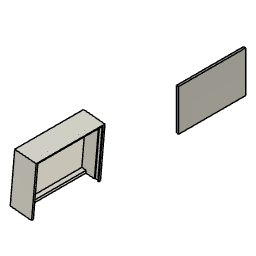
Configuration cool v3 (Autodesk Fusion 360 design; units mm, degrees)
Autodesk Fusion 360 part; units mm, degrees
note: some values were not read from the file. Set by a fixed rule: which sketch regions a step uses.
sketch "Sketch1" plane through (0, 0, 0) normal (1, 0, 0) x (0, 1, 0)
  line L0 (0, 0) -> (80, 0)
  line L1 (0, 0) -> (0, 60)
  line L2 (0, 60) -> (80, 60)
  line L3 (80, 60) -> (80, 0)
  dimension "d1" = 80
  constraint coincident L0.start L1.start
  constraint horizontal L0
  constraint perpendicular L0 L1
  constraint perpendicular L1 L2
  constraint perpendicular L0 L3
  measures "d1" distance of L0.start L0.end
extrude "Extrude1" add sketch "Sketch1" along normal blind 10 makes body 1
sketch "Sketch2" plane through (10, 0, 0) normal (1, 0, 0) x (0, 1, 0)
  line L0 (0, 0) -> (80, 0)
  line L1 (80, 0) -> (80, 60)
  line L2 (80, 60) -> (0, 60)
  line L3 (0, 60) -> (0, 0)
  line L4 (0, 60) -> (80, 60)
  line L5 (80, 0) -> (38, 0)
  line L6 (38, 58.7474) -> (2, 58.7474)
  line L7 (2, 58.7474) -> (2, 0)
  line L8 (0, 0) -> (2, 0)
  line L9 (38, 58.7474) -> (38, 0)
  constraint coincident L2.end L3.start
  constraint coincident L1.end L2.start
  constraint coincident L0.end L1.start
  constraint coincident L0 L5.end
  constraint perpendicular L1 L5
  constraint perpendicular L1 L6
  constraint coincident L0 L7.end
  constraint perpendicular L0 L7
  constraint coincident L0.start L3.end
  constraint perpendicular L5 L9
extrude "Extrude2" add sketch "Sketch2" along normal blind 15 contours L0 L1 L2 L3 L4 L5 L6 L7 L8 L9 bodies 1
sketch "Sketch3" plane through (10, 0, 0) normal (1, 0, 0) x (0, 1, 0)
  line L0 (2, 58.7474) -> (2, 0)
  line L1 (2, 0) -> (38, 0)
  line L2 (2, 0) -> (38, 0)
  line L3 (38, 2.9429) -> (2, 2.9429)
  line L4 (2, 0) -> (2, 2.9429)
  line L5 (38, 0) -> (38, 2.9429)
  line L6 (38, 0) -> (38, 58.7474)
  line L7 (38, 58.7474) -> (2, 58.7474)
  constraint coincident L0.end L1.start
  constraint coincident L1.end L2.end
  constraint coincident L0 L3.end
  constraint perpendicular L0 L3
  constraint perpendicular L3 L5
extrude "Extrude3" add sketch "Sketch3" along normal blind 5 contours L0 L1 L2 L3 L4 L5 L6 bodies 1
sketch "Sketch4" plane through (10, 0, 0) normal (1, 0, 0) x (0, 1, 0)
  line L0 (2, 2.9429) -> (38, 2.9429)
  line L1 (2, 58.7474) -> (2, 2.9429)
  line L2 (33.2817, -3.5012) -> (111.2817, -3.5012)
  line L3 (111.2817, -3.5012) -> (111.2817, 44.4988)
  line L4 (111.2817, 44.4988) -> (33.2817, 44.4988)
  line L5 (33.2817, 44.4988) -> (33.2817, -3.5012)
  line L6 (38, 2.9429) -> (38, 58.7474)
  line L7 (38, 58.7474) -> (2, 58.7474)
  dimension "d8" = 78
  dimension "d9" = 48
  constraint perpendicular L2 L3
  constraint perpendicular L3 L4
  constraint perpendicular L2 L5
  measures "d8" distance of L2.start L2.end
  measures "d9" distance of L2.end L3.end
extrude "Extrude4" add sketch "Sketch4" along normal blind 2 separate body contours L0 L4 L5 L6 | L0 L2 L3 L4 L5 L6 makes body 2
sketch "Sketch5" plane through (12, 0, 0) normal (1, 0, 0) x (0, 1, 0)
  line L0 (33.2817, 44.4988) -> (33.2817, -3.5012)
  line L1 (33.2817, -3.5012) -> (111.2817, -3.5012)
  line L2 (111.2817, -3.5012) -> (111.2817, 44.4988)
  line L3 (111.2817, 44.4988) -> (33.2817, 44.4988)
move_body "Move1" bodies 2 to x (1, 0, 0) y (0, 1, 0) z (0, 0, 1) at (15, -48, 2)
move_body "Move2" bodies 2 to x (1, 0, 0) y (0, 1, 0) z (0, 0, 1) at (-6, 0, 0)
sketch "Sketch6" plane through (21, 0, 0) normal (1, 0, 0) x (0, 1, 0)
  line L0 (-14.7183, 46.4988) -> (-14.7183, -1.5012)
  line L1 (-14.7183, -1.5012) -> (63.2817, -1.5012)
  line L2 (63.2817, -1.5012) -> (63.2817, 46.4988)
  line L3 (63.2817, 46.4988) -> (-14.7183, 46.4988)
move_body "Move3" bodies 2 to x (1, 0, 0) y (0, 1, 0) z (0, 0, 1) at (18, 0, 0)
sketch "Sketch7" plane through (39, 0, 0) normal (1, 0, 0) x (0, 1, 0)
  line L0 (-14.7183, 46.4988) -> (-14.7183, -1.5012)
  line L1 (-14.7183, -1.5012) -> (63.2817, -1.5012)
  line L2 (63.2817, -1.5012) -> (63.2817, 46.4988)
  line L3 (63.2817, 46.4988) -> (-14.7183, 46.4988)
sketch "Sketch8" plane through (39, 0, 0) normal (1, 0, 0) x (0, 1, 0)
  line L0 (-14.7183, 46.4988) -> (-14.7183, -1.5012)
  line L1 (-14.7183, -1.5012) -> (63.2817, -1.5012)
  line L2 (63.2817, -1.5012) -> (63.2817, 46.4988)
  line L3 (63.2817, 46.4988) -> (-14.7183, 46.4988)
move_body "Move4" bodies 2 to x (1, 0, 0) y (0, 1, 0) z (0, 0, 1) at (-1.5428, 1.8094, 0.4773)
move_body "Move5" bodies 2 to x (1, 0, 0) y (0, 1, 0) z (0, 0, 1) at (0, 10, 0)
move_body "Move6" bodies 2 to x (1, 0, 0) y (0, 1, 0) z (0, 0, 1) at (-15, 0, 0)
move_body "Move7" bodies 2 to x (1, 0, 0) y (0, 1, 0) z (0, 0, 1) at (0, -12, 0)
move_body "Move8" bodies 2 to x (1, 0, 0) y (0, 1, 0) z (0, 0, 1) at (10, 0, 0)
move_body "Move9" bodies 2 to x (1, 0, 0) y (0, 1, 0) z (0, 0, 1) at (0, 15, 5)
move_body "Move10" bodies 2 to x (1, 0, 0) y (0, 1, 0) z (0, 0, 1) at (0.5173, -18.9965, -0.6609)
move_body "Move11" bodies 2 to x (1, 0, 0) y (0, 1, 0) z (0, 0, 1) at (-13, 0, 0)
move_body "Move12" bodies 2 to x (1, 0, 0) y (0, 1, 0) z (0, 0, 1) at (0, 4, 0)
move_body "Move13" bodies 2 to x (1, 0, 0) y (0, 1, 0) z (0, 0, 1) at (10, 0, 0)
move_body "Move14" bodies 2 to x (1, 0, 0) y (0, 1, 0) z (0, 0, 1) at (0, 1, 0)
move_body "Move15" bodies 2 to x (1, 0, 0) y (0, 1, 0) z (0, 0, 1) at (21.2708, 41.4828, -21.4534)
move_body "Move16" bodies 2 to x (1, 0, 0) y (0, 1, 0) z (0, 0, 1) at (3.3836, 8.6688, 28.5327)
move_body "Move17" bodies 2 to x (1, 0, 0) y (0, 1, 0) z (0, 0, 1) at (-38.2468, 34.7717, -10.8051)
extrude "Extrude6" cut 1 faces at (16.6667, 38, 40.1459) along direction (0, 1, 0) blind 40 on bodies 1 bodies 1
extrude "Extrude7" add 1 faces at (25, 0.6667, 39.5825) along direction (1, 0, 0) blind 5 on bodies 1 bodies 1
sketch "Sketch10" plane through (0, 78, 0) normal (0, -1, 0) x (1, 0, 0)
  line L0 (15, 2.9429) -> (15, 0)
  line L1 (15, 0) -> (30, 0)
  line L2 (30, 0) -> (30, 58.7474)
  line L3 (30, 58.7474) -> (10, 58.7474)
  line L4 (10, 58.7474) -> (10, 2.9429)
  line L5 (10, 2.9429) -> (15, 2.9429)
move_body "Move18" bodies 2 to x (1, 0, 0) y (0, 1, 0) z (0, 0, 1) at (-1.1862, -16.387, -16.5072)
move_body "Move19" bodies 2 to x (1, 0, 0) y (0, 1, 0) z (0, 0, 1) at (16.0791, -7.3134, -20.0229)
move_body "Move20" bodies 2 to x (1, 0, 0) y (0, 1, 0) z (0, 0, 1) at (3.6083, -61.8453, 40.1901)
move_body "Move21" bodies 2 to x (1, 0, 0) y (0, 1, 0) z (0, 0, 1) at (0, 62.0564, 0.6442)
move_body "Move22" bodies 2 to x (1, 0, 0) y (0, 1, 0) z (0, 0, 1) at (0, 24.1549, -0.0402)
extrude "Extrude9" cut 1 faces at (0, 53.3333, 20) along direction (1, 0, 0) blind 5 on bodies 1 bodies 1
move_body "Move23" bodies 2 to x (1, 0, 0) y (0, 1, 0) z (0, 0, 1) at (29.6008, -117.5704, 12.6132)
move_face "MoveFace2" by (0.4671, 2.2152, 0.1877) 1 faces at (64.4841, -19.887, 48.4665) on bodies 2
move_body "Move24" bodies 2 to x (1, 0, 0) y (0, 1, 0) z (0, 0, 1) at (7.9958, 36.4984, 0.1207)
move_body "Move25" bodies 2 to x (1, 0, 0) y (0, 1, 0) z (0, 0, 1) at (-42.2189, -3.1812, -2.5327)
move_body "Move26" bodies 2 to x (1, 0, 0) y (0, 1, 0) z (0, 0, 1) at (-4.8101, 5.9711, -4.7452)
move_body "Move27" bodies 2 to x (1, 0, 0) y (0, 1, 0) z (0, 0, 1) at (0, 10, 0)
move_body "Move28" bodies 2 to x (1, 0, 0) y (0, 1, 0) z (0, 0, 1) at (0.9323, -4.3913, 0.3562)
move_body "Move29" bodies 2 to x (1, 0, 0) y (0, 1, 0) z (0, 0, 1) at (0, 85, 0)
move_body "Move30" bodies 2 to x (1, 0, 0) y (0, 1, 0) z (0, 0, 1) at (-33.607, -23.3616, -11.8616)
move_body "Move31" bodies 2 to x (1, 0, 0) y (0, 1, 0) z (0, 0, 1) at (38.2631, -58.5388, 14.0781)
move_body "Move32" bodies 2 to x (1, 0, 0) y (0, 1, 0) z (0, 0, 1) at (-2.622, 0.2288, 0.1219)
move_body "Move33" bodies 2 to x (1, 0, 0) y (0, 1, 0) z (0, 0, 1) at (0.162, -1.369, 0)
move_body "Move34" bodies 2 to x (1, 0, 0) y (0, 1, 0) z (0, 0, 1) at (60, 90, 0)
move_body "Move35" bodies 1 to x (-0.173648, 0, 0.984808) y (0, 1, 0) z (-0.984808, 0, -0.173648) at (30.4373, 0, 12.4387)
move_body "Move36" bodies 1 to x (0.173648, 0, 0.984808) y (0, 1, 0) z (-0.984808, 0, 0.173648) at (10.3453, 0, 19.7889)
move_body "Move37" bodies 1 to x (-0.939693, 0, 0.34202) y (0, 1, 0) z (-0.34202, 0, -0.939693) at (10.1419, 0, 75.882)
move_body "Move38" bodies 1 to x (-0.087156, 0, 0.996195) y (0, 1, 0) z (-0.996195, 0, -0.087156) at (52.2395, 0, 43.4919)
sketch "Sketch14" plane through (15.795, 0, -4.2323) normal (0.965926, 0, -0.258819) x (0, 1, 0)
  line L0 (0, 40.7267) -> (80, 40.7267)
  line L1 (80, 40.7267) -> (80, 65.7267)
  line L2 (80, 65.7267) -> (78, 65.7267)
  line L3 (78, 50.7267) -> (2, 50.7267)
  line L4 (2, 50.7267) -> (2, 65.7267) construction
  line L5 (2, 65.7267) -> (0, 65.7267)
  line L6 (0, 65.7267) -> (0, 40.7267)
  line L7 (80, 40.7267) -> (80, 65.7267)
  line L8 (0, 40.7267) -> (0, 65.7267)
  line L9 (2, 45.7267) -> (78, 45.7267)
  line L10 (78, 45.7267) -> (78, 65.7267) construction
  line L11 (78, 65.7267) -> (2, 65.7267)
  line L12 (2, 65.7267) -> (2, 45.7267) construction
  line L13 (78, 65.7267) -> (78, 64.7267)
  line L14 (78, 64.7267) -> (79, 64.7267)
  line L15 (0, 65.7267) -> (2, 65.7267)
  line L16 (79, 64.7267) -> (79, 60.7267)
  line L17 (79, 60.7267) -> (78, 60.7267)
  line L18 (40, 65.7267) -> (40, 60.7267) construction
  line L19 (40, 60.7267) -> (78, 60.7267)
  line L20 (40, 60.7267) -> (2, 60.7267)
  line L21 (1, 64.7267) -> (1, 60.7267)
  line L22 (1, 60.7267) -> (2, 60.7267)
  line L23 (2, 64.7267) -> (1, 64.7267)
  line L24 (2, 65.7267) -> (2, 64.7267)
  point P0 (78, 65.7267)
  point P1 (0, 65.7267)
  point P2 (2, 65.7267)
  dimension "d48" = 4
  dimension "d49" = 1
  dimension "d50" = 5
  constraint coincident P0 L2.end
  constraint perpendicular L14 L16
  constraint perpendicular L16 L17
  constraint midpoint L11 L18.start
  constraint perpendicular L11 L18
  constraint perpendicular L10 L19
  constraint symmetric P0 L18 P2
  constraint symmetric L13.end L18 L23.start
  constraint symmetric L14.end L18 L21.start
  constraint symmetric L16.end L18 L21.end
  constraint symmetric L17.end L18 L20.end
  constraint symmetric L19.start L18 L20.start
  measures "d48" distance of L14.end L16.end
  measures "d49" distance of L16.end L17.end
  measures "d50" distance of L18.start L18.end
extrude "Extrude10" cut sketch "Sketch14" against normal blind 59 contours L11 L13 L14 L16 L17 L19 L20 L21 L22 L23 L24 bodies 1
move_body "Move39" bodies 2 to x (1, 0, 0) y (0, 1, 0) z (0, 0, 1) at (4.1783, 25.0636, 29.9452)
move_body "Move40" bodies 1 to x (1, 0, 0) y (0, 1, 0) z (0, 0, 1) at (5.1764, 0, 19.3185)
move_body "Move41" bodies 1 to x (0, 0, -1) y (0, 1, 0) z (1, 0, 0) at (-22.913, 0, 85.9375)
move_body "Move42" bodies 1 to x (0.984808, 0, 0.173648) y (0, 1, 0) z (-0.173648, 0, 0.984808) at (10.4318, -18.6049, -52.6781)
named bodies: "main frame", "Cover"
